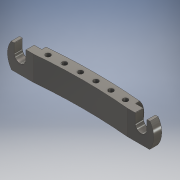
# Autodesk Inventor part: Ponte
Saved by Autodesk Inventor 2016 (Build 200138000, 138)
## iProperties
Created: 2018-12-06
Part Number: Ponte
Material: Generic
Document SubType Name: Sheet Metal
Designer: dqm_r
Density: 1 g/cm^3
Sheet Metal Rule: Default_mm
Appearance: Default
Author: dqm_r
Autodesk Inventor part; units mm, degrees
ref_plane "XZ Plane" through (0, 0, 0) normal (0, 1, 0) x (-1, 0, 0)
ref_plane "XY Plane" through (0, 0, 0) normal (0, 0, 1) x (1, 0, 0)
sketch "Sketch1" plane through (0, 0, 0) normal (0, 0, 1) x (1, 0, 0)
  arc A0 (32.28, 0) -> (-32.28, 0) centre (0, -346.5828) ccw
  line L0 (32.28, 0) -> (32.38, 0)
  line L1 (-32.28, 0) -> (-32.38, 0)
  point P0 (0, 0)
  dimension "d0" = 64.56
  dimension "d4" = 0.1
  dimension "d5" = 0.1
  constraints: 4 end point, 3 point on circle, 2 horizontal, 1 centre point, 1 other
  measures "d0" distance of L1.start A0.start
  measures "d4" distance of L0.start L0.end
  measures "d5" distance of L1.start L1.end
ref_plane "Work Plane2" through (32.28, 0, 0) normal (1, 0, 0) x (0, 1, 0)
sketch "Sketch2" plane through (32.28, 0, 0) normal (1, 0, 0) x (0, 1, 0)
  line L0 (-5.74, 8.5) -> (-5.74, -8.5)
  line L1 (1.76, -8.5) -> (5.74, -8.5)
  line L2 (2.76, 8.5) -> (-5.74, 8.5)
  line L3 (-5.74, -8.5) -> (1.76, -8.5)
  line L4 (1.76, -8.5) -> (2.76, -8.5)
  arc A0 (2.76, -8.5) -> (2.76, 8.5) centre (-7.8725, 0) ccw
  point P0 (0, 0)
  point P1 (0, 0)
  dimension "d7" = 17
  dimension "d8" = 11.48
  constraints: 10 end point, 2 point on circle, 1 centre point, 1 parallel, 1 perpendicular, 1 point on line, 1 vertical, 1 other
  measures "d7" distance of L0.start L0.end
  measures "d8" distance of L1.end L0.end
sweep "Sweep1" add profiles "Sketch2" path "Sketch1" keep normal constant yes path curves A0 L1
sketch "Sketch3" plane through (0, 0, 0) normal (0, 1, 0) x (-1, 0, 0)
  line L0 (32.38, -8.5) -> (32.38, 8.5) projected
  line L1 (47.6144, -8.5026) -> (32.38, -8.5)
  line L2 (32.38, 8.5) -> (37.7655, 8.5)
  line L3 (45.7655, 8.5) -> (47.88, 8.5)
  arc A0 (47.6144, -8.5026) -> (47.88, 8.5) centre (35.7156, 0.1866) ccw
  line L4 (45.7655, 2.1785) -> (45.7655, 8.5)
  line L5 (37.7655, 8.5) -> (37.7655, 2.1785)
  line L6 (32.38, 8.5) -> (37.7655, 8.5)
  line L7 (-32.1144, -8.5) -> (-32.1144, 8.5)
  arc A1 (37.7655, 2.1785) -> (45.7655, 2.1785) centre (41.7655, 2.1785) ccw
  line L8 (-32.28, -8.5) -> (-32.28, 8.5)
  line L9 (-47.6144, -8.5026) -> (-32.28, -8.5)
  line L10 (-32.28, 8.5) -> (-37.7655, 8.5)
  line L11 (-45.7655, 8.5) -> (-47.88, 8.5)
  arc A2 (-47.88, 8.5) -> (-47.6144, -8.5026) centre (-35.7156, 0.1866) ccw
  line L12 (-45.7655, 2.1785) -> (-45.7655, 8.5)
  line L13 (-37.7655, 8.5) -> (-37.7655, 2.1785)
  line L14 (-32.28, 8.5) -> (-37.7655, 8.5)
  arc A3 (-45.7655, 2.1785) -> (-37.7655, 2.1785) centre (-41.7655, 2.1785) ccw
  line L15 (-32.28, 8.5) -> (-32.28, -8.5) projected
  point P0 (0, 0)
  point P1 (-32.28, 0)
  dimension "d15" = 5.3855
  dimension "d17" = 2.1145
  constraints: 30 end point, 8 point on circle, 4 centre point, 2 midpoint, 2 tangent, 2 vertical, 1 horizontal, 1 other
  measures "d15" distance of L0.end L2.end
  measures "d17" distance of L3.start L3.end
extrude "Extrusion1" add sketch "Sketch3" against normal up to surface (5.74 mm away)
sketch "Sketch5" plane through (0, -343.8228, 8.5) normal (0, 0, 1) x (1, 0, 0)
  circle A0 centre (-26.88, 342.505) radius 2.5004 projected
  circle A1 centre (-26.88, 342.505) radius 2.5004
  circle A2 centre (-16.1789, 343.1458) radius 2.5004 projected
  circle A3 centre (-16.1789, 343.1458) radius 2.5004
  circle A4 centre (-5.4631, 343.4539) radius 2.5004 projected
  circle A5 centre (-5.4631, 343.4539) radius 2.5004
  circle A6 centre (5.2571, 343.429) radius 2.5004 projected
  circle A7 centre (5.2571, 343.429) radius 2.5004
  circle A8 centre (15.9713, 343.0711) radius 2.5004 projected
  circle A9 centre (15.9713, 343.0711) radius 2.5004
  circle A10 centre (26.6693, 342.3806) radius 2.5004 projected
  circle A11 centre (26.6693, 342.3806) radius 2.5004
  point P0 (0, 343.8228)
  constraints: 6 centre point, 6 coincident, 1 other
hole "Hole2" at (-26.88, -1.3178, 8.5) at (-16.1789, -0.677, 8.5) at (-5.4631, -0.3689, 8.5) at (5.2571, -0.3938, 8.5) at (15.9713, -0.7517, 8.5) at (26.6693, -1.4422, 8.5) direction (0, 0, -1) diameter 3.5 end through all
sketch "Sketch7" plane through (0, -343.8228, -8.5) normal (0, 0, -1) x (-1, 0, 0)
  circle A0 centre (-15.9713, 343.0711) radius 2.5004 projected
  circle A1 centre (-26.6693, 342.3806) radius 2.5004 projected
  circle A2 centre (-5.2571, 343.429) radius 2.5004 projected
  circle A3 centre (5.4631, 343.4539) radius 2.5004 projected
  circle A4 centre (16.1789, 343.1458) radius 2.5004 projected
  circle A5 centre (26.88, 342.505) radius 2.5004 projected
  point P0 (0, 343.8228)
extrude "Extrusion3" cut sketch "Sketch7" against normal blind 4
sketch "Sketch8" plane through (-32.38, -5.54, -8.5) normal (0, 0, -1) x (-1, 0, 0)
  circle A0 centre (-5.5, 4.2222) radius 2.5004 projected
  arc A1 (-0.0907, 0) -> (-64.66, 0.0009) centre (-32.38, -346.7828) ccw projected
  circle A2 centre (-59.0493, 4.0978) radius 1.75 projected
  arc A3 (-5.5, 4.2222) -> (-59.0493, 4.0978) centre (-31.6727, -254.8368) ccw construction
  arc A4 (-1.2142, 3.4513) -> (-63.3198, 3.3083) centre (-31.6727, -254.8368) ccw
  arc A5 (-1.2142, 4.0554) -> (-63.3198, 3.9128) centre (-31.6727, -254.8368) ccw
  line L0 (-64.4944, 5.34) -> (-64.4944, 0.0162) projected
  line L1 (-64.4944, 0.0162) -> (-64.4944, 5.34)
  line L2 (-1.2142, 4.0438) -> (-1.2142, 4.0554)
  line L3 (-1.2142, 4.0438) -> (-1.2142, 3.4513)
  line L4 (-63.3198, 3.9088) -> (-63.3198, 3.9128)
  line L5 (-63.3198, 3.3083) -> (-63.3198, 3.9088)
  point P0 (-32.38, 5.54)
  point P1 (0, 5.34)
  dimension "d67" = 0.3
  dimension "d68" = 0.3
  constraints: 10 end point, 7 point on circle, 3 centre point, 2 collinear, 2 point on line, 2 vertical
  measures "d67" radial gap between concentric circles of A3 A4
  measures "d68" radial gap between concentric circles of A3 A5
extrude "Extrusion4" cut sketch "Sketch8" against normal blind 2 contours A0 A4 A5 | A0 A5 L2 L3 A4 | A0 A4 A2 A5 | A2 A4 A5 | A2 A4 L5 L4 A5
chamfer "Chamfer1" distance 0.3 angle 45 17 edges at (21.3399, -0.633, -8.5) (21.3154, -1.2331, -8.5) (10.6151, -0.5456, -8.5) (10.6278, 0.0544, -8.5) (30.0549, -1.5205, -8.5) (30.022, -2.1208, -8.5) (30.9398, -1.6292, -8.5) (30.9398, -1.9314, -8.5) (-0.1028, -0.2997, -8.5) (-0.1014, 0.3003, -8.5) (-10.8318, 0.1043, -8.5) (-10.8218, -0.4958, -8.5) (-21.5469, -0.5334, -8.5) (-21.5252, -1.1336, -8.5) (-30.2416, -1.9814, -8.5) (-30.2731, -1.3811, -8.5) (-31.1658, -1.7867, -8.5)
fillet "Fillet2" radius 0.2 6 edges at (31.2398, -1.7133, -8.5) (30.1283, -2.4356, -8.5) (30.044, -1.2171, -8.5) (-31.4658, -1.8222, -8.5) (-30.4116, -1.095, -8.5) (-30.3486, -2.2957, -8.5)
fillet "Fillet5" radius 0.2 17 edges at (-50.4476, 0, -0.0435) (-39.9972, 0, -8.5013) (-41.7655, 0, -1.8215) (-45.7655, 0, 5.3393) (-37.7655, 0, 5.3393) (-35.0727, 0, 8.5) (-37.7655, -2.87, 8.5) (-45.7655, -2.87, 8.5) (39.9472, 0, -8.5013) (50.4476, 0, -0.0435) (46.8227, 0, 8.5) (41.7655, 0, -1.8215) (37.7655, 0, 5.3393) (45.7655, 0, 5.3393) (35.0227, 0, 8.5) (45.7655, -2.87, 8.5) (37.7655, -2.87, 8.5)
equation "\"d64\" = Thickness"
equation "\"BendRadius\" = Thickness"
equation "\"BendReliefWidth\" = Thickness"
equation "\"BendReliefDepth\" = 0.5 * Thickness"
equation "\"CornerReliefSize\" = 4 * Thickness"
equation "\"MinimumRemnant\" = 2 * Thickness"
equation "\"TransitionRadius\" = BendRadius"
equation "\"JacobiRadiusSize\" = BendRadius"
equation "\"GapSize\" = Thickness"
equation "\"Thickness\" = 0.5"
body "Solid1"
